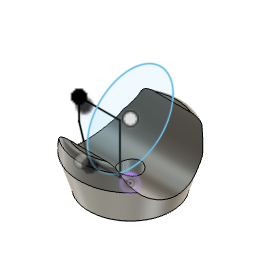
Saddles v3 (Autodesk Fusion 360 design; units mm, degrees)
Autodesk Fusion 360 part; units mm, degrees
sketch "Sketch5" plane through (0, 0, 0) normal (0, 1, 0) x (1, 0, 0)
  line L0 (-4, 0) -> (-12.75, 0)
  line L1 (-12.75, 0) -> (-12.75, 2)
  line L2 (-4, 0) -> (-4, -19)
  line L3 (0, 0) -> (-4, 0)
  line L4 (-19.75, -17) -> (-19.75, -10.75)
  line L5 (-4, -19) -> (-17.75, -19)
  arc A0 (-19.75, -17) -> (-17.75, -19) centre (-17.75, -17) ccw
  line L6 (-12.75, 2) -> (-15.0157, 2)
  line L7 (-15.9698, 1.2993) -> (-19.75, -10.75)
  arc A1 (-15.0157, 2) -> (-15.9698, 1.2993) centre (-15.0157, 1) ccw
  point P0 (-18.75, 1.9185)
  point P1 (-19.75, -19)
  point P2 (-15.75, 2)
  dimension "d103" = 12.75
  dimension "d112" = 19
  dimension "d113" = 4
  dimension "d123" = 2
  dimension "d126" = 2
  dimension "d127" = 3
  dimension "d129" = 17
  dimension "d130" = 17.75
  dimension "d131" = 8.25
  dimension "d132" = 1
  constraint horizontal L0
  constraint perpendicular L0 L1
  constraint perpendicular L0 L2
  constraint coincident L3.start origin
  constraint perpendicular L2 L3
  constraint perpendicular L4 L5
  constraint coincident P1 L5
  constraint coincident L4 P1
  constraint tangent L5 A0
  constraint tangent L4 A0
  constraint perpendicular L1 L6
  constraint coincident P2 L7
  constraint coincident P2 L6
  constraint tangent L7 A1
  constraint tangent L6 A1
  measures "d103" distance of L3.start L0.end
  measures "d112" distance of L0.start L2.end
  measures "d113" distance of L3.start L0.start
  measures "d123" radius of A0
  measures "d126" distance of L0.end L1.end
  measures "d127" distance of L1.end P2
  measures "d129" vertical distance of L3.start A0.centre
  measures "d130" horizontal distance of L3.start A0.centre
  measures "d131" vertical distance of L2.end L4.end
  measures "d132" radius of A1
sketch "Sketch6" plane through (0, 0, 0) normal (1, 0, 0) x (0, 1, 0)
  circle A0 centre (0, 21.5) radius 16.5
  dimension "d115" = 33
  dimension "d118" = 21.5
  measures "d115" diameter of A0
  measures "d118" distance of A0.centre origin
revolve "Revolve3" add sketch "Sketch5" angle 360 about axis through (0, 0, 1.75) along (0, 0, 1)
extrude "Extrude5" cut sketch "Sketch6" along normal mid plane 66
equation "terminalTubeDiameter = 25 mm"
equation "crossTubeDiameter = 33 mm"
equation "boltHoleDiameter = 8 mm"
equation "d103 = ( terminalTubeDiameter + 0.5 mm ) / 2"
equation "d112 = ( crossTubeDiameter / 2 ) + 2.5 mm"
equation "d113 = boltHoleDiameter / 2"
equation "d115 = crossTubeDiameter"
equation "d118 = ( crossTubeDiameter / 2 ) + 5 mm"
equation "d129 = ( crossTubeDiameter / 2 ) + 0.5 mm"
equation "d130 = ( ( crossTubeDiameter + 0.5 mm ) / 2 ) + 1 mm"
equation "d131 = crossTubeDiameter / 4"
equation "d134 = max(crossTubeDiameter; terminalTubeDiameter)"
